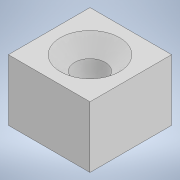
# Autodesk Inventor part: Тестовая модель (винты и гайки)
Saved by Autodesk Inventor 2020 (Build 240168000, 168)
## iProperties
Created: 2021-04-05
Part Number: Тестовая модель (винты и гайки)
Material: Типовые
Document SubType Name: Modeling
Designer: Антон
Density: 1 g/cm^3
Appearance: По умолчанию
Author: Антон
Autodesk Inventor part; units mm, degrees
ref_plane "YZ Plane" through (0, 0, 0) normal (1, 0, 0) x (0, 1, 0)
ref_plane "XZ Plane" through (0, 0, 0) normal (0, 1, 0) x (-1, 0, 0)
ref_plane "XY Plane" through (0, 0, 0) normal (0, 0, 1) x (1, 0, 0)
sketch "Эскиз1" plane through (0, 0, 0) normal (0, 1, 0) x (-1, 0, 0)
  line L0 (0, 0) -> (8, 0)
  line L1 (8, 0) -> (8, -8)
  line L2 (8, -8) -> (0, -8)
  line L3 (0, -8) -> (0, 0)
  dimension "d0" = 8
  dimension "d1" = 8
  constraints: 8 end point, 2 parallel, 1 horizontal, 1 perpendicular
  measures "d0" distance of L1.end L2.end
  measures "d1" distance of L0.end L1.end
extrude "Выдавливание1" add sketch "Эскиз1" along normal blind 6
sketch "Эскиз2" plane through (0, 6, 0) normal (0, 1, 0) x (1, 0, 0)
  line L0 (-8, 0) -> (0, 0) projected
  line L1 (-4, 0) -> (-4, 8)
  line L2 (0, 8) -> (-8, 8) projected
  point P0 (-4, 4)
  constraints: 3 midpoint, 2 end point
hole "Отверстие1" at (-4, 6, -4) direction (0, -1, 0) diameter 3 end through all countersink diameter 5.8 countersink angle 90
sketch "Эскиз3" plane through (0, 0, 0) normal (0, -1, 0) x (1, 0, 0)
  circle A0 centre (-4, -4) radius 1.5 projected
  line L0 (-5.6166, -6.8) -> (-7.2332, -4)
  line L1 (-7.2332, -4) -> (-5.6166, -1.2)
  line L2 (-5.6166, -1.2) -> (-2.3834, -1.2)
  line L3 (-2.3834, -1.2) -> (-0.7668, -4)
  line L4 (-0.7668, -4) -> (-2.3834, -6.8)
  line L5 (-2.3834, -6.8) -> (-5.6166, -6.8)
  point P0 (0, 0)
  dimension "d12" = 5.6
  constraints: 12 end point, 1 coincident, 13 other
  measures "d12" distance between parallel lines of L5 L2
extrude "Выдавливание2" cut sketch "Эскиз3" against normal blind 2.6
